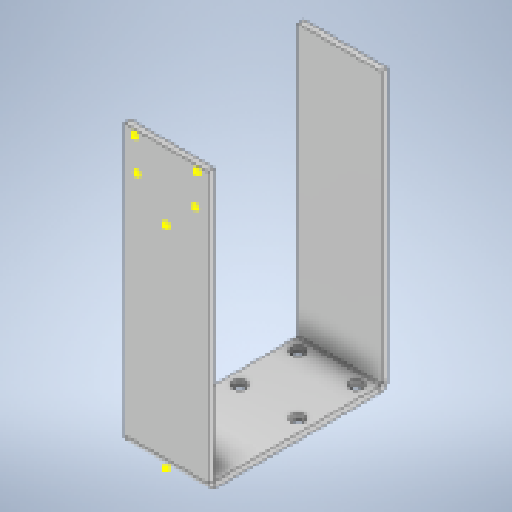
# Autodesk Inventor part: axis_25_top_frame
Saved by Autodesk Inventor 2025.2 (Build 292293000, 293)
## iProperties
Created: 2025-06-30
Part Number: axis_25_top_frame
Material: Aluminum 6061-AHC
Document SubType Name: Sheet Metal
Designer: LG
Density: 2.7 g/cm^3
Sheet Metal Rule: Default_mm
Appearance: Aluminum - Dark
Author: LG
Autodesk Inventor part; units mm, degrees
ref_plane "YZ Plane" through (0, 0, 0) normal (1, 0, 0) x (0, 1, 0)
ref_plane "XZ Plane" through (0, 0, 0) normal (0, 1, 0) x (-1, 0, 0)
ref_plane "XY Plane" through (0, 0, 0) normal (0, 0, 1) x (1, 0, 0)
sketch "Sketch1" plane through (0, 0, 0) normal (0, 1, 0) x (-1, 0, 0)
  line L0 (10.07, 20.05) -> (-10.07, 20.05)
  line L1 (-10.07, 20.05) -> (-10.07, -20.05)
  line L2 (-10.07, -20.05) -> (10.07, -20.05)
  line L3 (10.07, -20.05) -> (10.07, 20.05)
  point P0 (0, 0)
  dimension "d0" = 40.1
  dimension "d1" = 20.14
  dimension "d2" = 10.07
  dimension "d3" = 20.05
  measures "d0" distance of L2.end L0.start
  measures "d1" distance of L1.end L2.end
  measures "d2" distance from line of point (0, 0) L3
  measures "d3" distance from line of point (0, 0) L2
extrude "Plate1" add sketch "Sketch1" along normal blind 1.5
sketch "Sketch2" plane through (10.07, 0, 21.55) normal (0, 0, -1) x (-1, 0, 0)
  line L0 (20.14, 0) -> (0, 0)
  line L1 (0, 0) -> (0, 66.74)
  line L2 (0, 66.74) -> (20.14, 66.74)
  line L3 (20.14, 66.74) -> (20.14, 0)
  constraints: 8 end point
edge flange "Flange1" height 66.74 angle 90 thickness 1.5 bend radius 0.31 thickness toward (0, 0, -1) relief straight relief width 1.5 relief depth 0.75 corner gap 0.31 corner form 0 edges at (0, 1.5, 20.05) (0, 1.5, -20.05) wall of the first edge with corners at (-10.07, 0, 21.55) (10.07, 0, 21.55) (10.07, 66.74, 21.55) (-10.07, 66.74, 21.55)
bend "Bend1"
corner "Corner1"
sketch "Sketch7" plane through (10.07, 66.74, -21.55) normal (0, 0, -1) x (-1, 0, 0)
  circle A0 centre (2.545, -2.5) radius 0.7835
  circle A1 centre (17.595, -2.5) radius 0.7835
  circle A2 centre (2.545, -22.5) radius 0.7835
  circle A3 centre (17.595, -22.5) radius 0.7835
  circle A4 centre (2.545, -37.6) radius 0.7835
  circle A5 centre (17.595, -37.6) radius 0.7835
  point P0 (10.07, -66.74)
  constraints: 6 centre point, 12 other
hole "Hole4" at (7.525, 64.24, -21.55) at (-7.525, 64.24, -21.55) at (7.525, 44.24, -21.55) at (-7.525, 44.24, -21.55) at (7.525, 29.14, -21.55) at (-7.525, 29.14, -21.55) direction (0, 0, 1) diameter 2.1 depth 1.5
sketch "Sketch8" plane through (-10.07, 66.74, 21.55) normal (0, 0, 1) x (1, 0, 0)
  circle A0 centre (2, -2) radius 0.7835
  circle A1 centre (18.14, -2) radius 0.7835
  circle A2 centre (2.07, -16.9) radius 0.7835
  circle A3 centre (18.07, -16.9) radius 0.7835
  circle A4 centre (17.07, -30.12) radius 0.7835
  circle A5 centre (3.07, -30.12) radius 0.7835
  circle A6 centre (10.07, -37.42) radius 0.7835
  point P0 (10.07, -66.74)
  constraints: 7 centre point, 14 other
hole "Hole5" at (-8.07, 64.74, 21.55) at (8.07, 64.74, 21.55) at (-8, 49.84, 21.55) at (8, 49.84, 21.55) at (-7, 36.62, 21.55) at (7, 36.62, 21.55) at (0, 29.32, 21.55) direction (0, 0, -1) diameter 2.1 depth 1.5
sketch "Sketch9" plane through (-10.07, 66.74, 21.55) normal (0, 0, 1) x (1, 0, 0)
  circle A0 centre (10.07, -10) radius 6
  point P0 (10.07, -66.74)
  constraints: 1 centre point, 2 other
extrude "Cut2" cut sketch "Sketch9" against normal blind 1.5
sketch "Sketch10" plane through (10.07, 66.74, -21.55) normal (0, 0, -1) x (-1, 0, 0)
  circle A0 centre (10.07, -10) radius 6
  point P0 (10.07, -66.74)
  constraints: 1 centre point, 2 other
extrude "Cut3" cut sketch "Sketch10" against normal blind 1.5
sketch "Sketch11" plane through (0, 0, 0) normal (0, -1, 0) x (1, 0, 0)
  circle A0 centre (7, 9) radius 1.55
  circle A1 centre (7, -9) radius 1.55
  circle A2 centre (-7, 9) radius 1.55
  circle A3 centre (-7, -9) radius 1.55
  point P0 (0, 0)
  dimension "d56" = 3.1
  dimension "d57" = 7
  dimension "d58" = 9
  dimension "d59" = 3.1
  dimension "d60" = 9
  dimension "d61" = 7
  dimension "d62" = 3.1
  dimension "d63" = 9
  dimension "d64" = 7
  dimension "d65" = 3.1
  dimension "d66" = 7
  dimension "d67" = 9
  constraints: 4 centre point
  measures "d56" diameter of A0
  measures "d57" horizontal distance of point (0, 0) A0.centre
  measures "d58" vertical distance of point (0, 0) A0.centre
  measures "d59" diameter of A1
  measures "d60" vertical distance of point (0, 0) A1.centre
  measures "d61" horizontal distance of point (0, 0) A1.centre
  measures "d62" diameter of A2
  measures "d63" vertical distance of point (0, 0) A2.centre
  measures "d64" horizontal distance of point (0, 0) A2.centre
  measures "d65" diameter of A3
  measures "d66" horizontal distance of point (0, 0) A3.centre
  measures "d67" vertical distance of point (0, 0) A3.centre
extrude "Cut4" cut sketch "Sketch11" against normal blind 1.5
equation "\"d43\" = Thickness"
equation "\"d50\" = Thickness"
equation "\"d52\" = Thickness"
equation "\"d54\" = Thickness"
equation "\"d68\" = Thickness"
equation "\"d4\" = Thickness"
equation "\"d5\" = BendReliefWidth"
equation "\"d6\" = BendReliefDepth"
equation "\"d7\" = MinimumRemnant"
equation "\"d8\" = TransitionRadius"
equation "\"d11\" = BendRadius"
equation "\"d12\" = CornerReliefSize"
equation "\"d13\" = GapSize"
equation "\"d14\" = JacobiRadiusSize"
equation "\"BendReliefWidth\" = Thickness"
equation "\"BendReliefDepth\" = 0.5 * Thickness"
equation "\"CornerReliefSize\" = 4 * Thickness"
equation "\"MinimumRemnant\" = 2 * Thickness"
equation "\"TransitionRadius\" = BendRadius"
equation "\"JacobiRadiusSize\" = BendRadius"
equation "\"GapSize\" = Thickness"
equation "\"Thickness\" = 1.5"
equation "\"BendRadius\" = 0.31"
body "Solid1"
